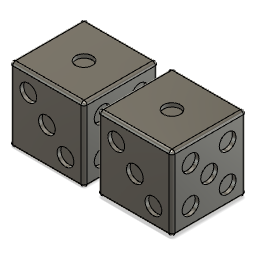
dice v1 (Autodesk Fusion 360 design; units mm, degrees)
Autodesk Fusion 360 part; units mm, degrees
sketch "Sketch1" plane through (0, 0, 0) normal (0, 1, 0) x (1, 0, 0)
  line L0 (50.8, -50.8) -> (-50.8, -50.8)
  line L1 (-50.8, -50.8) -> (-50.8, 50.8)
  line L2 (-50.8, 50.8) -> (50.8, 50.8)
  line L3 (50.8, 50.8) -> (50.8, -50.8)
  line L4 (50.8, -50.8) -> (-50.8, 50.8) construction
  line L5 (-50.8, -50.8) -> (50.8, 50.8) construction
  dimension "d1" = 101.6
  dimension "d2" = 101.6
  constraint horizontal L0
  constraint perpendicular L0 L1
  constraint parallel L0 L2
  constraint parallel L1 L3
  constraint coincident L4 origin
  constraint coincident L5 origin
  measures "d1" distance of L1.end L2.end
  measures "d2" distance of L0.end L1.end
extrude "Extrude1" add sketch "Sketch1" along normal mid plane 101.6 makes body 1
sketch "Sketch2" plane through (0, 50.8, 0) normal (0, 1, 0) x (-1, 0, 0)
  line L0 (-50.8, -50.8) -> (50.8, -50.8)
  line L1 (50.8, -50.8) -> (50.8, 50.8)
  line L2 (50.8, 50.8) -> (-50.8, 50.8)
  line L3 (-50.8, 50.8) -> (-50.8, -50.8)
  circle A0 centre (0, 0) radius 11.43
  dimension "d5" = 22.86
  constraint coincident A0.centre origin
  measures "d5" diameter of A0
extrude "Extrude2" cut sketch "Sketch2" against normal blind 5.08 contours A0 bodies 1
sketch "Sketch3" plane through (0, 0, 50.8) normal (0, 0, 1) x (1, 0, 0)
  line L0 (-50.8, -50.8) -> (50.8, -50.8)
  line L1 (50.8, -50.8) -> (50.8, 50.8)
  line L2 (50.8, 50.8) -> (-50.8, 50.8)
  line L3 (-50.8, 50.8) -> (-50.8, -50.8)
sketch "Sketch4" plane through (0, 0, 50.8) normal (0, 0, 1) x (1, 0, 0)
  circle A0 centre (0, 0) radius 11.43
  line L0 (-50.8, 50.8) -> (0, 0) construction
  line L1 (0, 0) -> (50.8, -50.8) construction
  circle A1 centre (-25.4, 25.4) radius 11.43
  circle A2 centre (25.4, -25.4) radius 11.43
  dimension "d8" = 22.86
  constraint coincident A0.centre L0.end
  constraint parallel L0 L1
  constraint midpoint L0 A1.centre
  constraint midpoint L1 A2.centre
  constraint equal A0 A1
  constraint equal A0 A2
  measures "d8" diameter of A0
extrude "Extrude3" cut sketch "Sketch4" against normal blind 5.08 bodies 1
sketch "Sketch5" plane through (50.8, 0, 0) normal (1, 0, 0) x (0, 0, -1)
  line L0 (50.8, -50.8) -> (50.8, 50.8)
  line L1 (50.8, 50.8) -> (-50.8, 50.8)
  line L2 (-50.8, 50.8) -> (-50.8, -50.8)
  line L3 (-50.8, -50.8) -> (50.8, -50.8)
  line L4 (-50.8, 50.8) -> (0, 0) construction
  line L5 (0, 0) -> (50.8, -50.8) construction
  line L6 (50.8, 50.8) -> (0, 0) construction
  line L7 (0, 0) -> (-50.8, -50.8) construction
  circle A0 centre (0, 0) radius 11.43
  circle A1 centre (-25.4, 25.4) radius 11.43
  circle A2 centre (25.4, 25.4) radius 11.43
  circle A3 centre (25.4, -25.4) radius 11.43
  circle A4 centre (-25.4, -25.4) radius 11.43
  dimension "d11" = 22.86
  constraint coincident L1.end L2.start
  constraint coincident L4.end L5.start
  constraint coincident L0.start L3.end
  constraint coincident L0.end L1.start
  constraint coincident L2.end L3.start
  constraint midpoint L4 A1.centre
  constraint midpoint L6 A2.centre
  constraint midpoint L5 A3.centre
  constraint midpoint L7 A4.centre
  constraint equal A0 A1
  constraint equal A0 A2
  constraint equal A0 A3
  constraint equal A0 A4
  measures "d11" diameter of A0
extrude "Extrude4" cut sketch "Sketch5" against normal blind 5.08 contours A0 | A1 | A2 | A3 | A4 bodies 1
sketch "Sketch6" plane through (0, 0, -50.8) normal (0, 0, -1) x (-1, 0, 0)
  line L0 (50.8, -50.8) -> (50.8, 50.8)
  line L1 (50.8, 50.8) -> (-50.8, 50.8)
  line L2 (-50.8, 50.8) -> (-50.8, -50.8)
  line L3 (-50.8, -50.8) -> (50.8, -50.8)
  line L4 (-50.8, 50.8) -> (0, 0) construction
  line L5 (0, 0) -> (50.8, -50.8) construction
  line L6 (50.8, 50.8) -> (0, 0) construction
  line L7 (0, 0) -> (-50.8, -50.8) construction
  circle A0 centre (-25.4, 25.4) radius 11.43
  circle A1 centre (25.4, 25.4) radius 11.43
  circle A2 centre (25.4, -25.4) radius 11.43
  circle A3 centre (-25.4, -25.4) radius 11.43
  dimension "d25" = 22.86
  constraint coincident L1.end L2.start
  constraint coincident L4.end L5.start
  constraint coincident L0.start L3.end
  constraint coincident L0.end L1.start
  constraint coincident L2.end L3.start
  constraint midpoint L4 A0.centre
  constraint midpoint L6 A1.centre
  constraint midpoint L5 A2.centre
  constraint midpoint L7 A3.centre
  constraint equal A2 A3
  constraint equal A1 A2
  constraint equal A0 A1
  measures "d25" diameter of A3
extrude "Extrude5" cut sketch "Sketch6" against normal blind 5.08 contours A0 | A1 | A2 | A3 bodies 1
sketch "Sketch7" plane through (-50.8, 0, 0) normal (-1, 0, 0) x (0, 0, 1)
  line L0 (50.8, -50.8) -> (50.8, 50.8)
  line L1 (50.8, 50.8) -> (-50.8, 50.8)
  line L2 (-50.8, 50.8) -> (-50.8, -50.8)
  line L3 (-50.8, -50.8) -> (50.8, -50.8)
  line L4 (-50.8, 50.8) -> (0, 0) construction
  line L5 (0, 0) -> (50.8, -50.8) construction
  circle A0 centre (-25.4, 25.4) radius 12.7
  circle A1 centre (25.4, -25.4) radius 11.43
  dimension "d17" = 25.4
  dimension "d18" = 22.86
  constraint coincident L1.end L2.start
  constraint coincident L4.end L5.start
  constraint coincident L0.start L3.end
  constraint midpoint L4 A0.centre
  constraint midpoint L5 A1.centre
  measures "d17" diameter of A0
  measures "d18" diameter of A1
extrude "Extrude6" cut sketch "Sketch7" against normal blind 5.08 contours A0 | A1 bodies 1
sketch "Sketch8" plane through (0, -50.8, 0) normal (0, -1, 0) x (1, 0, 0)
  line L0 (-50.8, -50.8) -> (50.8, -50.8)
  line L1 (50.8, -50.8) -> (50.8, 50.8)
  line L2 (50.8, 50.8) -> (-50.8, 50.8)
  line L3 (-50.8, 50.8) -> (-50.8, -50.8)
  line L4 (-50.8, 50.8) -> (0, 0) construction
  line L5 (0, 0) -> (50.8, -50.8) construction
  line L6 (50.8, 50.8) -> (0, 0) construction
  line L7 (-50.8, -50.8) -> (0, 0) construction
  line L8 (-50.8, 0) -> (0, 0) construction
  line L9 (50.8, 0) -> (0, 0) construction
  circle A0 centre (-25.4, 25.4) radius 11.43
  circle A1 centre (-25.4, 0) radius 11.43
  circle A2 centre (-25.4, -25.4) radius 11.43
  circle A3 centre (25.4, -25.4) radius 11.43
  circle A4 centre (25.4, 0) radius 11.43
  circle A5 centre (25.4, 25.4) radius 11.43
  dimension "d21" = 22.86
  constraint coincident L2.end L3.start
  constraint coincident L4.end L5.start
  constraint coincident L0.end L1.start
  constraint coincident L1.end L2.start
  constraint coincident L0.start L3.end
  constraint midpoint L3 L8.start
  constraint midpoint L1 L9.start
  constraint midpoint L4 A0.centre
  constraint midpoint L8 A1.centre
  constraint midpoint L7 A2.centre
  constraint midpoint L5 A3.centre
  constraint midpoint L9 A4.centre
  constraint midpoint L6 A5.centre
  constraint equal A4 A5
  constraint equal A3 A4
  constraint equal A0 A5
  constraint equal A1 A4
  constraint equal A2 A5
  measures "d21" diameter of A5
extrude "Extrude7" cut sketch "Sketch8" against normal blind 5.08 contours A0 | A1 | A2 | A3 | A4 | A5 bodies 1
fillet "Fillet1" radius 4.064 12 edges at (0, 50.8, 50.8) (-50.8, 50.8, 0) (-50.8, 0, 50.8) (50.8, 50.8, 0) (0, 50.8, -50.8) (50.8, 0, -50.8) (-50.8, 0, -50.8) (50.8, 0, 50.8) (0, -50.8, -50.8) (-50.8, -50.8, 0) (50.8, -50.8, 0) (0, -50.8, 50.8) on bodies 1
copy_body "CopyPasteBodies1" bodies 1 makes body 2
move_body "Move1" bodies 2 to x (1, 0, 0) y (0, 1, 0) z (0, 0, 1) at (-120.2418, -2.2242, 0)
equation "d1 = Dicesize"
equation "d2 = Dicesize"
equation "d3 = Dicesize"
equation "d5 = DivotDia"
equation "d6 = -DivotDepth"
equation "d8 = DivotDia"
equation "d9 = -DivotDepth"
equation "d11 = DivotDia"
equation "d12 = -DivotDepth"
equation "d15 = -DivotDepth"
equation "d18 = DivotDia"
equation "d19 = -DivotDepth"
equation "d21 = DivotDia"
equation "Dicesize = 4 in"
equation "DivotDia = Dicesize / 4 - 0.1 in"
equation "DivotDepth = Dicesize / 20"
equation "d25 = DivotDia"
equation "d26 = -DivotDepth"
equation "d29 = Dicesize / 25"
